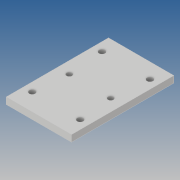
# Autodesk Inventor part: attache_exterieur
Saved by Autodesk Inventor 2019 (Build 230136000, 136)
## iProperties
Created: 2020-07-07
Part Number: attache_exterieur
Material: Générique
Document SubType Name: Modeling
Designer: Theo
Density: 1 g/cm^3
Appearance: Par défaut
Author: Theo
Autodesk Inventor part; units mm, degrees
ref_plane "YZ Plane" through (0, 0, 0) normal (1, 0, 0) x (0, 1, 0)
ref_plane "XZ Plane" through (0, 0, 0) normal (0, 1, 0) x (-1, 0, 0)
ref_plane "XY Plane" through (0, 0, 0) normal (0, 0, 1) x (1, 0, 0)
sketch "Esquisse1" plane through (0, 0, 0) normal (0, 1, 0) x (-1, 0, 0)
  line L0 (0, 0) -> (-60, 0)
  line L1 (-60, 0) -> (-60, 94)
  line L2 (-60, 94) -> (0, 94)
  line L3 (0, 94) -> (0, 0)
  dimension "d0" = 60
  dimension "d1" = 94
  constraints: 8 end point, 2 parallel, 1 horizontal, 1 perpendicular
  measures "d0" distance of L0.start L0.end
  measures "d1" distance of L2.end L0.start
extrude "Extrusion1" add sketch "Esquisse1" along normal blind 6
sketch "Esquisse2" plane through (0, 6, 0) normal (0, 1, 0) x (1, 0, 0)
  line L0 (0, -94) -> (60, -94) projected
  line L1 (60, 0) -> (0, 0) projected
  line L2 (0, 0) -> (0, -94) projected
  line L3 (60, -94) -> (60, 0) projected
  point P0 (8, -78)
  point P1 (52, -78)
  point P2 (52, -14)
  point P3 (8, -14)
  dimension "d4" = 16
  dimension "d5" = 14
  dimension "d6" = 8
  dimension "d7" = 8
  constraints: 2 horizontal alignment, 2 vertical alignment
  measures "d4" distance from line of L0 point (8, -78)
  measures "d5" distance from line of L1 point (8, -14)
  measures "d6" distance from line of L2 point (8, -78)
  measures "d7" distance from line of L3 point (52, -78)
hole "Perçage1" at (8, 6, 78) at (52, 6, 78) at (52, 6, 14) at (8, 6, 14) direction (0, -1, 0) diameter 5.5 end through all clearance for "Vis d'assemblage à tête hexagonale ISO 24017" size "M5" standard "ISO"
sketch "Esquisse4" plane through (0, 0, 0) normal (0, -1, 0) x (1, 0, 0)
  line L0 (0, 94) -> (0, 0) projected
  line L1 (60, 0) -> (60, 94) projected
  point P0 (11, 47)
  point P1 (49, 47)
  point P2 (0, 47)
  dimension "d15" = 11
  dimension "d16" = 11
  constraints: 2 horizontal alignment, 1 midpoint
  measures "d15" distance from line of L0 point (11, 47)
  measures "d16" distance from line of L1 point (49, 47)
hole "Perçage2" at (11, 0, 47) at (49, 0, 47) direction (0, 1, 0) diameter 5 end through all countersink diameter 10 countersink angle 90
equation "\"d16\" = d15"
